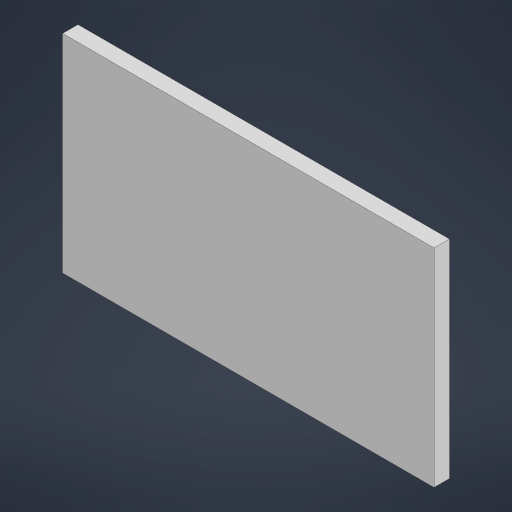
# Autodesk Inventor part: TV
Saved by Autodesk Inventor 2024.2 (Build 282272000, 272)
## iProperties
Created: 2025-08-11
Part Number: TV
Material: Generic
Document SubType Name: Modeling
Designer: Luca
Density: 1 g/cm^3
Appearance: Default
Author: Luca
Autodesk Inventor part; units mm, degrees
ref_plane "YZ Plane" through (0, 0, 0) normal (1, 0, 0) x (0, 1, 0)
ref_plane "XZ Plane" through (0, 0, 0) normal (0, 1, 0) x (-1, 0, 0)
ref_plane "XY Plane" through (0, 0, 0) normal (0, 0, 1) x (1, 0, 0)
sketch "Sketch1" plane through (0, 0, 0) normal (0, 0, 1) x (1, 0, 0)
  line L0 (-725, -405) -> (725, -405)
  line L1 (725, -405) -> (725, 405)
  line L2 (725, 405) -> (-725, 405)
  line L3 (-725, 405) -> (-725, -405)
  line L4 (-725, -405) -> (725, 405) construction
  line L5 (725, -405) -> (-725, 405) construction
  point P0 (0, 0)
  dimension "d0" = 1450
  dimension "d1" = 810
  constraints: 12 end point, 2 midpoint, 2 parallel, 1 horizontal, 1 perpendicular
  measures "d0" distance of L2.end L1.end
  measures "d1" distance of L1.end L0.end
extrude "Extrusion1" add sketch "Sketch1" along normal blind 60
body "Solid1"
